start switch_v1 (Autodesk Fusion 360 design; units mm, degrees)
Autodesk Fusion 360 part; units mm, degrees
sketch "Esquisse1" plane through (0, 0, 0) normal (0, 0, 1) x (1, 0, 0)
  line L0 (8, 6.5) -> (-8, 6.5)
  line L1 (-8, 6.5) -> (-8, -6.5)
  line L2 (-8, -6.5) -> (8, -6.5)
  line L3 (8, -6.5) -> (8, 6.5)
  line L4 (8, 6.5) -> (-8, -6.5) construction
  line L5 (-8, 6.5) -> (8, -6.5) construction
  line L6 (-10, -8.5) -> (10, -8.5)
  line L7 (10, -8.5) -> (10, 8.5)
  line L8 (10, 8.5) -> (-10, 8.5)
  line L9 (-10, 8.5) -> (-10, -8.5)
  circle A0 centre (-5, -3.5) radius 2
  dimension "d1" = 16
  dimension "d2" = 13
  dimension "d3" = 2
  dimension "d15" = 4
  dimension "d16" = 3
  dimension "d18" = 3
  constraint horizontal L0
  constraint perpendicular L0 L1
  constraint parallel L0 L2
  constraint parallel L1 L3
  constraint coincident L4 origin
  constraint coincident L5 origin
  measures "d1" distance of L1.end L2.end
  measures "d2" distance of L0.end L1.end
  measures "d15" diameter of A0
  measures "d16" distance of L1 A0.centre
  measures "d18" distance of L2 A0.centre
extrude "Extrusion1" add sketch "Esquisse1" along normal blind 32 contours L6 L7 L8 L9
extrude "Extrusion2" add sketch "Esquisse1" along normal blind 3 contours L0 L1 L2 L3
sketch "Esquisse2" plane through (0, -8.5, 0) normal (0, -1, 0) x (1, 0, 0)
  line L0 (-10, 0) -> (10, 0)
  line L1 (10, 0) -> (10, 32)
  line L2 (10, 32) -> (-10, 32)
  line L3 (-10, 32) -> (-10, 0)
  line L4 (16, 32) -> (-16, 32)
  line L5 (-16, 32) -> (-16, 0)
  line L6 (-16, 0) -> (16, 0)
  line L7 (16, 0) -> (16, 32)
  line L8 (16, 32) -> (-16, 0) construction
  line L9 (-16, 32) -> (16, 0) construction
  line L10 (-10, 0) -> (10, 0)
  circle A0 centre (13, 29) radius 1.7
  line L11 (0, 16) -> (16, 16) construction
  line L12 (0, 16) -> (0, 32) construction
  circle A1 centre (13, 3) radius 1.7
  circle A2 centre (-13, 3) radius 1.7
  circle A3 centre (-13, 29) radius 1.7
  point P0 (0, 16)
  dimension "d8" = 6
  dimension "d9" = 6
  dimension "d10" = 3.4
  dimension "d11" = 3
  dimension "d12" = 3
  constraint horizontal L4
  constraint perpendicular L4 L5
  constraint parallel L4 L6
  constraint parallel L5 L7
  constraint coincident L8 P0
  constraint coincident L9 P0
  constraint collinear L2 L4
  constraint collinear L6 L10
  constraint coincident P0 L11.start
  constraint midpoint L7 L11.end
  constraint midpoint L4 L12.end
  constraint symmetric A0 L11 A1
  constraint symmetric A0 L12 A3
  constraint symmetric L12 A1 A2
  measures "d8" distance of L1 L7
  measures "d9" distance of L3 L5
  measures "d10" diameter of A0
  measures "d11" distance of L7 A0.centre
  measures "d12" distance of L4 A0.centre
extrude "Extrusion3" add sketch "Esquisse2" against normal blind 3 contours L3 L4 L5 L6 | L1 L4 L6 L7
equation "d9 = d8"
equation "d18 = d16"
